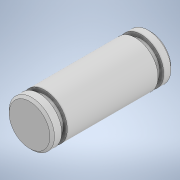
# Autodesk Inventor part: Peça30
Saved by Autodesk Inventor 2021 (Build 250183000, 183)
## iProperties
Created: 2021-07-21
Part Number: Peça30
Material: Genérico
Document SubType Name: Modeling
Designer: Giovanni
Density: 1 g/cm^3
Appearance: Padrão
Author: Giovanni
Autodesk Inventor part; units mm, degrees
ref_plane "YZ Plane" through (0, 0, 0) normal (1, 0, 0) x (0, 1, 0)
ref_plane "XZ Plane" through (0, 0, 0) normal (0, 1, 0) x (-1, 0, 0)
ref_plane "XY Plane" through (0, 0, 0) normal (0, 0, 1) x (1, 0, 0)
sketch "Esboço1" plane through (0, 0, 0) normal (0, 0, 1) x (1, 0, 0)
  circle A0 centre (0, 0) radius 3
  dimension "d0" = 6
  constraints: 1 centre point, 1 coincident
  measures "d0" diameter of A0
extrude "Extrusão1" add sketch "Esboço1" along normal mid plane 16
sketch "Esboço2" plane through (0, 0, 0) normal (1, 0, 0) x (0, 1, 0)
  line L0 (3.25, -6) -> (2.5, -6)
  line L1 (2.5, -6) -> (2.5, -6.75)
  line L2 (2.5, -6.75) -> (3.25, -6.75)
  line L3 (3.25, -6.75) -> (3.25, -6)
  line L4 (3.1313, 6.75) -> (2.5, 6.75)
  line L5 (2.5, 6.75) -> (2.5, 6)
  line L6 (2.5, 6) -> (3.1313, 6)
  line L7 (3.1313, 6) -> (3.1313, 6.75)
  line L8 (0, 0) -> (0, -8)
  line L9 (-3, -8) -> (3, -8) projected
  dimension "d3" = 5
  dimension "d4" = 6.5
  dimension "d5" = 6
  dimension "d6" = 0.75
  dimension "d7" = 6
  dimension "d8" = 0.75
  constraints: 18 end point, 4 parallel, 2 horizontal, 2 perpendicular, 1 midpoint
  measures "d3" diameter of L1 L8
  measures "d4" diameter of L3 L8
  measures "d5" vertical distance of L0.start L8.start
  measures "d6" distance of L2.end L0.start
  measures "d7" vertical distance of L6.end L8.start
  measures "d8" distance of L6.end L4.start
revolve "Revolução1" cut sketch "Esboço2" angle 360 about axis through (0, 0, 0) along (0, 0, -1)
chamfer "Chanfro1" distance 0.3 angle 45 2 edges at (-3, 0, 8) (-3, 0, -8)
